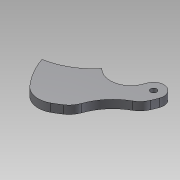
# Autodesk Inventor part: launcher.latch
Saved by Autodesk Inventor 2011 (Build 150239000, 239)
## iProperties
Created: 2011-02-22
Part Number: launcher.latch
Document SubType Name: Modeling
Designer: Casey
Density: 1 g/cm^3
Author: Casey
Autodesk Inventor part; units mm, degrees
ref_plane "YZ Plane" through (0, 0, 0) normal (1, 0, 0) x (0, 1, 0)
ref_plane "XZ Plane" through (0, 0, 0) normal (0, 1, 0) x (-1, 0, 0)
ref_plane "XY Plane" through (0, 0, 0) normal (0, 0, 1) x (1, 0, 0)
sketch "Sketch1" plane through (0, 0, 0) normal (0, 0, 1) x (1, 0, 0)
  circle A0 centre (46.0449, -16.759) radius 4 construction
  spline S0 degree 3 poles (32.2129, 20.8318) (30.525, 21.8832) (29.0415, 23.2334) (25.9174, 26.8655) (24.5253, 29.2164) (23.4072, 31.3618) knots 0 0 0 0 0.391133 0.391133 0.939024 0.939024 0.939024 0.939024 construction
  arc A1 (50.7434, -18.4691) -> (41.3465, -15.0489) centre (46.0449, -16.759) ccw
  circle A2 centre (46.0449, -16.759) radius 1.5
  arc A3 (5.4493, -30.9044) -> (24.0394, -20.1714) centre (0, 0) ccw
  arc A4 (26.086, -47.2813) -> (50.7434, -18.4691) centre (0, 0) ccw
  arc A5 (40.5335, -17.1182) -> (41.3465, -15.0489) centre (0, 0) ccw
  circle A6 centre (0, 0) radius 49 construction
  line L0 (46.0449, -16.759) -> (0, 0) construction
  line L1 (0, 0) -> (49, 0) construction
  line L2 (5.4493, -30.9044) -> (0, 0) construction
  line L3 (24.0394, -20.1714) -> (0, 0) construction
  line L4 (24.0394, -20.1714) -> (24.8935, -20.8881)
  line L5 (0, 0) -> (15.6906, -27.1769) construction
  arc A7 (24.8935, -20.8881) -> (40.5335, -17.1182) centre (31.3214, -13.2277) ccw
  arc A8 (5.4493, -30.9044) -> (13.7408, -45.1235) centre (46.0449, -16.759) ccw
  arc A9 (13.7408, -45.1235) -> (26.086, -47.2813) centre (21.2552, -38.5255) ccw
  point P0 (33.706, -28.2827)
  dimension "d2" = 62.7624
  dimension "d3" = 10
  dimension "d4" = 3
  dimension "d5" = 8
  dimension "d42" = 98
  dimension "d45" = 20
  dimension "d46" = 40
  dimension "d47" = 20
  dimension "d48" = 60
  dimension "d49" = 10
  dimension "d51" = 10
  constraints: 18 point on circle, 12 end point, 10 centre point, 6 tangent, 5 coincident, 2 concentric, 1 collinear, 1 horizontal, 1 point on line, 3 other
  measures "d2" diameter of A3
  measures "d3" diameter of A1
  measures "d4" diameter of A2
  measures "d5" diameter of A0
  measures "d42" diameter of A6
  measures "d45" angle of L0 L1
  measures "d46" angle of L2 L3
  measures "d47" angle of L5 L2
  measures "d48" angle of L1 L5
  measures "d49" radius of A7
  measures "d51" radius of A9
extrude "Extrusion1" add sketch "Sketch1" along normal blind 4
sketch "Sketch10" plane through (0, 0, 4) normal (0, 0, 1) x (1, 0, 0)
  arc A0 (26.086, -47.2813) -> (50.7434, -18.4691) centre (0, 0) ccw projected
  arc A1 (47.7831, -25.1551) -> (33.0704, -42.689) centre (57.4533, -48.2091) ccw
  arc A2 (40.5335, -17.1182) -> (41.3465, -15.0489) centre (0, 0) ccw projected
  line L0 (57.4533, -48.2091) -> (0, 0) construction
  line L1 (0, 0) -> (52.518, 0) construction
  dimension "d54" = 40
  dimension "d55" = 25
  dimension "d56" = 75
  constraints: 4 end point, 4 point on circle, 1 centre point, 1 horizontal
  measures "d54" angle of L1 L0
  measures "d55" radius of A1
  measures "d56" distance of L0.start L0.end
extrude "Extrusion9" cut sketch "Sketch10" against normal blind 10
fillet "Fillet8" radius 10 2 edges at (47.7831, -25.1551, 2) (33.0704, -42.689, 2)
equation "\"d51\" = d49"
body "Solid1"
